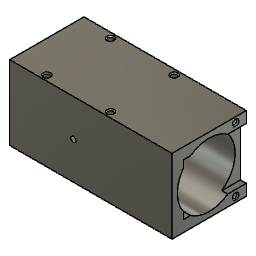
Task2 v2 (Autodesk Fusion 360 design; units mm, degrees)
Autodesk Fusion 360 part; units mm, degrees
sketch "Sketch1" plane through (0, 0, 0) normal (0, 1, 0) x (1, 0, 0)
  line L0 (38.25, 17.5) -> (-38.25, 17.5)
  line L1 (-38.25, 17.5) -> (-38.25, -17.5)
  line L2 (-38.25, -17.5) -> (38.25, -17.5)
  line L3 (38.25, -17.5) -> (38.25, 17.5)
  line L4 (38.25, 17.5) -> (-38.25, -17.5) construction
  line L5 (-38.25, 17.5) -> (38.25, -17.5) construction
  dimension "d1" = 76.5
  dimension "d2" = 35
  constraint horizontal L0
  constraint perpendicular L0 L1
  constraint parallel L0 L2
  constraint parallel L1 L3
  constraint coincident L4 origin
  constraint coincident L5 origin
  measures "d1" distance of L1.end L2.end
  measures "d2" distance of L0.end L1.end
extrude "Extrude1" add sketch "Sketch1" along normal blind 35
sketch "Sketch2" plane through (38.25, 0, 0) normal (1, 0, 0) x (0, 0, -1)
  line L0 (-17.5, 0) -> (17.5, 0)
  line L1 (17.5, 0) -> (17.5, 35)
  line L2 (17.5, 35) -> (-17.5, 35)
  line L3 (-17.5, 35) -> (-17.5, 0)
  circle A0 centre (0, 17.5) radius 15
  line L4 (0, 17.5) -> (17.5, 17.5) construction
  line L5 (17.5, 17.5) -> (17.5, 29.7)
  line L6 (17.5, 29.7) -> (-12, 29.7)
  line L7 (-12, 29.7) -> (-12, 5.3)
  line L8 (-12, 5.3) -> (17.5, 5.3)
  line L9 (17.5, 5.3) -> (17.5, 17.5)
  circle A1 centre (12.5, 32.5) radius 1.25 construction
  circle A2 centre (12.5, 2.5) radius 1.25 construction
  dimension "d5" = 30
  dimension "d6" = 17.5
  dimension "d7" = 17.5
  dimension "d8" = 12.2
  dimension "d9" = 29.5
  dimension "d10" = 24.4
  dimension "d11" = 2.5
  dimension "d12" = 2.5
  dimension "d13" = 5
  dimension "d14" = 2.5
  dimension "d15" = 5
  dimension "d16" = 2.5
  constraint coincident A0.centre L4.start
  constraint midpoint L1 L4.end
  constraint perpendicular L4 L5
  constraint perpendicular L5 L6
  constraint perpendicular L0 L7
  constraint coincident L1 L8.end
  constraint perpendicular L1 L8
  measures "d5" diameter of A0
  measures "d6" distance of L3 A0.centre
  measures "d7" distance of L0 A0.centre
  measures "d8" distance of L4.end L5.end
  measures "d9" distance of L5.end L6.end
  measures "d10" distance of L6.end L7.end
  measures "d11" diameter of A1
  measures "d12" distance of L2 A1.centre
  measures "d13" distance of L1 A1.centre
  measures "d14" diameter of A2
  measures "d15" distance of L1 A2.centre
  measures "d16" distance of L0 A2.centre
extrude "Extrude2" cut sketch "Sketch2" against normal blind 25.5 contours A0 L6 L7 L8 | A0 L8 | A0 L6 | A0 L7
extrude "Extrude3" cut sketch "Sketch2" against normal blind 2.75 contours L1 A0 L5 L6 L8 L9 | A0 L7 L8 | A0 L6 L7
sketch "Sketch3" plane through (-38.25, 0, 0) normal (-1, 0, 0) x (0, 0, 1)
  line L0 (-17.5, 0) -> (17.5, 0)
  line L1 (17.5, 0) -> (17.5, 35)
  line L2 (17.5, 35) -> (-17.5, 35)
  line L3 (-17.5, 35) -> (-17.5, 0)
  circle A0 centre (0, 17.5) radius 15
  line L4 (13.7179, 3.7821) -> (13.7179, 31.2179) construction
  line L5 (13.7179, 31.2179) -> (-13.7179, 31.2179) construction
  line L6 (-13.7179, 31.2179) -> (-13.7179, 3.7821) construction
  line L7 (-13.7179, 3.7821) -> (13.7179, 3.7821) construction
  circle A1 centre (-13.7179, 31.2179) radius 1.5
  circle A2 centre (13.7179, 31.2179) radius 1.5
  circle A3 centre (13.7179, 3.7821) radius 1.5
  circle A4 centre (-13.7179, 3.7821) radius 1.5
  point P0 (0, 17.5)
  dimension "d21" = 30
  dimension "d22" = 17.5
  dimension "d23" = 17.5
  dimension "d24" = 19.4
  dimension "d25" = 3
  dimension "d26" = 3
  dimension "d27" = 3
  dimension "d28" = 3
  constraint coincident P0 A0.centre
  constraint horizontal L5
  constraint coincident L5.end L6.start
  constraint coincident L4.end L5.start
  constraint coincident L4.start L7.end
  constraint coincident L6.end L7.start
  measures "d21" diameter of A0
  measures "d22" distance of L2 P0
  measures "d23" distance of L1 P0
  measures "d24" distance of L4.start P0
  measures "d25" diameter of A1
  measures "d26" diameter of A2
  measures "d27" diameter of A3
  measures "d28" diameter of A4
extrude "Extrude4" cut sketch "Sketch3" against normal blind 10 contours A0
sketch "Sketch4" plane through (-28.25, 0, 0) normal (-1, 0, 0) x (0, 0, 1)
  circle A0 centre (0, 17.5) radius 15
  circle A1 centre (0, 17.5) radius 12.5
  dimension "d31" = 25
  constraint concentric A0 A1
  measures "d31" diameter of A1
extrude "Extrude5" cut sketch "Sketch4" against normal blind 41 contours A1
sketch "Sketch5" plane through (0, 0, 17.5) normal (0, 0, 1) x (1, 0, 0)
  line L0 (-38.25, 0) -> (38.25, 0)
  line L1 (38.25, 0) -> (38.25, 35)
  line L2 (38.25, 35) -> (-38.25, 35)
  line L3 (-38.25, 35) -> (-38.25, 0)
  line L4 (-38.25, 17.5) -> (-8.25, 17.5) construction
  line L5 (-8.25, 17.5) -> (11.75, 17.5) construction
  circle A0 centre (-8.25, 17.5) radius 1.25
  circle A1 centre (11.75, 17.5) radius 2.5
  dimension "d34" = 30
  dimension "d35" = 20
  dimension "d36" = 2.5
  dimension "d37" = 5
  constraint midpoint L3 L4.start
  constraint perpendicular L3 L4
  constraint perpendicular L3 L5
  constraint coincident L4.end L5.start
  constraint coincident L5.end A1.centre
  measures "d34" distance of L4.start L4.end
  measures "d35" distance of L4.end L5.end
  measures "d36" diameter of A0
  measures "d37" diameter of A1
extrude "Extrude6" cut sketch "Sketch5" against normal blind 35 contours A0
extrude "Extrude7" cut sketch "Sketch5" along normal blind -20 and the other way blind 35 contours A1
sketch "Sketch6" plane through (0, 35, 0) normal (0, 1, 0) x (-1, 0, 0)
  line L0 (-38.25, 17.5) -> (-38.25, -17.5)
  line L1 (-38.25, -17.5) -> (38.25, -17.5)
  line L2 (38.25, -17.5) -> (38.25, 17.5)
  line L3 (38.25, 17.5) -> (-38.25, 17.5)
  circle A0 centre (23.25, -15) radius 1.5
  circle A1 centre (-6.75, -15) radius 1.5
  circle A2 centre (23.25, 15) radius 1.5
  circle A3 centre (-6.75, 15) radius 1.5
  dimension "d44" = 3
  dimension "d45" = 15
  dimension "d46" = 2.5
  dimension "d49" = -30
  dimension "d50" = 30
  measures "d44" diameter of A0
  measures "d45" distance of L2 A0.centre
  measures "d46" distance of L1 A0.centre
sketch "Sketch7" plane through (0, 0, 0) normal (0, -1, 0) x (1, 0, 0)
  line L0 (38.25, -17.5) -> (38.25, 17.5)
  line L1 (38.25, 17.5) -> (-38.25, 17.5)
  line L2 (-38.25, 17.5) -> (-38.25, -17.5)
  line L3 (-38.25, -17.5) -> (38.25, -17.5)
  circle A0 centre (-23.25, 15) radius 1.5
  circle A1 centre (6.75, 15) radius 1.5
  circle A2 centre (-23.25, -15) radius 1.5
  circle A3 centre (6.75, -15) radius 1.5
  dimension "d51" = 3
  dimension "d52" = 2.5
  dimension "d53" = 15
  dimension "d56" = 30
  dimension "d57" = -30
  measures "d51" diameter of A0
  measures "d52" distance of L1 A0.centre
  measures "d53" distance of L2 A0.centre
hole "Hole1" at (-38.25, 31.2179, 13.7179) at (-38.25, 31.2179, -13.7179) at (-38.25, 3.7821, -13.7179) at (-38.25, 3.7821, 13.7179) direction (1, 0, 0) diameter 2.5 depth 7 tip angle 118 countersink diameter 3.5 countersink angle 90
hole "Hole2" at (-23.25, 35, 15) at (6.75, 35, 15) at (6.75, 35, -15) at (-23.25, 35, -15) direction (0, -1, 0) diameter 2.5 depth 7 tip angle 118 countersink diameter 3.5 countersink angle 90
hole "Hole3" at (-23.25, 0, 15) at (-23.25, 0, -15) at (6.75, 0, -15) at (6.75, 0, 15) direction (0, 1, 0) diameter 2.5 depth 7 tip angle 118 countersink diameter 3.5 countersink angle 90
hole "Hole4" at (38.25, 32.5, -12.5) at (38.25, 2.5, -12.5) direction (-1, 0, 0) diameter 2.05 depth 5 tip angle 118 countersink diameter 3.05 countersink angle 90
equation "d24 = ( 38.8 / 2 ) * 1 mm"
equation "d46 = ( 5 / 2 ) * 1 mm"
equation "d52 = ( 5 / 2 ) * 1 mm"
